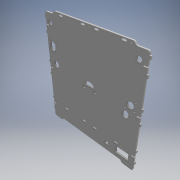
# Autodesk Inventor part: painel traseiro
Saved by Autodesk Inventor 2016 (Build 200138000, 138)
## iProperties
Created: 2016-08-08
Part Number: painel traseiro
Material: Generic
Document SubType Name: Modeling
Designer: Waldo
Density: 1 g/cm^3
Appearance: Default
Author: Waldo
Autodesk Inventor part; units mm, degrees
ref_plane "YZ Plane" through (0, 0, 0) normal (1, 0, 0) x (0, 1, 0)
ref_plane "XZ Plane" through (0, 0, 0) normal (0, 1, 0) x (-1, 0, 0)
ref_plane "XY Plane" through (0, 0, 0) normal (0, 0, 1) x (1, 0, 0)
sketch "Sketch1" plane through (0, 0, 0) normal (0, 1, 0) x (-1, 0, 0)
  line L0 (85.8953, -106.3896) -> (75.8953, -106.3896)
  line L1 (75.8953, -112.5896) -> (85.8953, -112.5896)
  line L2 (-145.1047, -106.3896) -> (-155.1047, -106.3896)
  line L3 (-155.1047, -112.5896) -> (-145.1047, -112.5896)
  line L4 (-54.6047, -106.3896) -> (-64.6047, -106.3896)
  line L5 (-64.6047, -112.5896) -> (-54.6047, -112.5896)
  line L6 (-4.6047, -106.3896) -> (-14.6047, -106.3896)
  line L7 (-14.6047, -112.5896) -> (-4.6047, -112.5896)
  line L8 (85.8953, 235.6104) -> (75.8953, 235.6104)
  line L9 (75.8953, 229.4104) -> (85.8953, 229.4104)
  line L10 (-145.1047, 235.6104) -> (-155.1047, 235.6104)
  line L11 (-155.1047, 229.4104) -> (-145.1047, 229.4104)
  line L12 (-54.6047, 235.6104) -> (-64.6047, 235.6104)
  line L13 (-64.6047, 229.4104) -> (-54.6047, 229.4104)
  line L14 (-4.6047, 235.6104) -> (-14.6047, 235.6104)
  line L15 (-14.6047, 229.4104) -> (-4.6047, 229.4104)
  line L16 (153.7371, 188.86) -> (147.2451, 188.86)
  line L17 (153.7371, 205.76) -> (153.7371, 188.86)
  line L18 (157.8955, 207.3098) -> (155.2869, 207.3098)
  line L19 (157.8955, 217.3104) -> (157.8955, 207.3098)
  line L20 (155.2869, 217.3104) -> (157.8955, 217.3104)
  line L21 (153.7371, 223.1102) -> (153.7371, 218.8602)
  line L22 (121.7453, 229.1102) -> (147.7371, 229.1102)
  line L23 (112.0224, 235.9739) -> (115.234, 232.1465)
  line L24 (105.511, 239.0102) -> (-174.7203, 239.0102)
  line L25 (-181.2317, 235.9739) -> (-184.4433, 232.1465)
  line L26 (-190.9547, 229.1102) -> (-216.9547, 229.1102)
  line L27 (-222.9547, 223.1102) -> (-222.9547, 218.8602)
  line L28 (-224.5045, 217.3104) -> (-227.1045, 217.3104)
  line L29 (-227.1045, 217.3104) -> (-227.1045, 207.3098)
  line L30 (-227.1045, 207.3098) -> (-224.5045, 207.3098)
  line L31 (-222.9547, 205.76) -> (-222.9547, 188.86)
  line L32 (-216.4542, 188.86) -> (-222.9547, 188.86)
  line L33 (-213.3942, 190.0596) -> (-214.9445, 190.0596)
  line L34 (-211.8813, 188.6771) -> (-211.8813, 188.8463)
  line L35 (-211.8813, 185.7741) -> (-211.8813, 185.9434)
  line L36 (-214.9445, 184.5607) -> (-213.3942, 184.5607)
  line L37 (-222.9547, 185.7604) -> (-216.4542, 185.7604)
  line L38 (-222.9547, 185.7604) -> (-222.9547, 168.8609)
  line L39 (-227.1127, 167.3111) -> (-224.5045, 167.3111)
  line L40 (-227.1127, 157.3107) -> (-227.1127, 167.3111)
  line L41 (-224.5045, 157.3107) -> (-227.1127, 157.3107)
  line L42 (-222.9547, 155.7609) -> (-222.9547, 65.5609)
  line L43 (-224.5045, 64.0111) -> (-227.1045, 64.0111)
  line L44 (-227.1045, 64.0111) -> (-227.1045, 54.0107)
  line L45 (-227.1045, 54.0107) -> (-224.5045, 54.0107)
  line L46 (-222.9547, 35.5607) -> (-222.9547, 52.4609)
  line L47 (-216.4542, 35.5607) -> (-222.9547, 35.5607)
  line L48 (-213.3942, 36.7603) -> (-214.9445, 36.7603)
  line L49 (-211.8813, 35.3778) -> (-211.8813, 35.547)
  line L50 (-211.8813, 32.4748) -> (-211.8813, 32.6441)
  line L51 (-214.9445, 31.2614) -> (-213.3942, 31.2614)
  line L52 (-222.9547, 32.4611) -> (-216.4542, 32.4611)
  line L53 (-222.9547, 15.5609) -> (-222.9547, 32.4611)
  line L54 (-227.1045, 14.0111) -> (-224.5045, 14.0111)
  line L55 (-227.1045, 4.0107) -> (-227.1045, 14.0111)
  line L56 (-224.5045, 4.0107) -> (-227.1045, 4.0107)
  line L57 (-222.9547, 2.4609) -> (-222.9547, -87.7398)
  line L58 (-224.5045, -89.2896) -> (-227.1045, -89.2896)
  line L59 (-227.1045, -89.2896) -> (-227.1045, -99.29)
  line L60 (-227.1045, -99.29) -> (-224.5045, -99.29)
  line L61 (-222.9547, -117.74) -> (-222.9547, -100.8398)
  line L62 (-216.4542, -117.74) -> (-222.9547, -117.74)
  line L63 (-213.3942, -116.5404) -> (-214.9445, -116.5404)
  line L64 (-211.8813, -117.9229) -> (-211.8813, -117.7537)
  line L65 (-211.8813, -120.8259) -> (-211.8813, -120.6566)
  line L66 (-214.9445, -122.0393) -> (-213.3942, -122.0393)
  line L67 (-222.9547, -120.8396) -> (-216.4542, -120.8396)
  line L68 (-222.9547, -137.7398) -> (-222.9547, -120.8396)
  line L69 (-227.1045, -139.2896) -> (-224.5045, -139.2896)
  line L70 (-227.1045, -149.29) -> (-227.1045, -139.2896)
  line L71 (-224.5045, -149.29) -> (-227.1045, -149.29)
  line L72 (-222.9547, -150.8398) -> (-222.9547, -174.9898)
  line L73 (-216.9547, -180.9898) -> (-184.9547, -180.9898)
  line L74 (-178.4433, -177.9535) -> (-174.2511, -172.9575)
  line L75 (100.8221, -170.9898) -> (-170.0314, -170.9898)
  line L76 (109.234, -177.9535) -> (105.0418, -172.9575)
  line L77 (147.7371, -180.9898) -> (115.7453, -180.9898)
  line L78 (153.7371, -150.8398) -> (153.7371, -174.9898)
  line L79 (155.2869, -149.29) -> (157.8955, -149.29)
  line L80 (157.8955, -149.29) -> (157.8955, -139.2896)
  line L81 (157.8955, -139.2896) -> (155.2869, -139.2896)
  line L82 (153.7371, -137.7398) -> (153.7371, -120.8396)
  line L83 (147.2451, -120.8396) -> (153.7371, -120.8396)
  line L84 (144.1849, -122.0393) -> (145.7353, -122.0393)
  line L85 (142.672, -120.6566) -> (142.672, -120.8259)
  line L86 (142.672, -117.7537) -> (142.672, -117.9229)
  line L87 (145.7354, -116.5404) -> (144.1849, -116.5404)
  line L88 (153.7371, -117.74) -> (147.2451, -117.74)
  line L89 (153.7371, -117.74) -> (153.7371, -100.8398)
  line L90 (157.8955, -99.29) -> (155.2869, -99.29)
  line L91 (157.8955, -89.2896) -> (157.8955, -99.29)
  line L92 (155.2869, -89.2896) -> (157.8955, -89.2896)
  line L93 (153.7371, 2.4609) -> (153.7371, -87.7398)
  line L94 (155.2869, 4.0107) -> (157.8955, 4.0107)
  line L95 (157.8955, 4.0107) -> (157.8955, 14.0111)
  line L96 (157.8955, 14.0111) -> (155.2869, 14.0111)
  line L97 (153.7371, 15.5609) -> (153.7371, 32.4611)
  line L98 (147.2451, 32.4611) -> (153.7371, 32.4611)
  line L99 (144.1849, 31.2614) -> (145.7353, 31.2614)
  line L100 (142.672, 32.6441) -> (142.672, 32.4748)
  line L101 (142.672, 35.547) -> (142.672, 35.3778)
  line L102 (145.7354, 36.7603) -> (144.1849, 36.7603)
  line L103 (153.7371, 35.5607) -> (147.2451, 35.5607)
  line L104 (153.7371, 35.5607) -> (153.7371, 52.4609)
  line L105 (157.8873, 54.0107) -> (155.2869, 54.0107)
  line L106 (157.8873, 64.0111) -> (157.8873, 54.0107)
  line L107 (155.2869, 64.0111) -> (157.8873, 64.0111)
  line L108 (153.7371, 155.7609) -> (153.7371, 65.5609)
  line L109 (155.2869, 157.3107) -> (157.8873, 157.3107)
  line L110 (157.8873, 157.3107) -> (157.8873, 167.3111)
  line L111 (157.8873, 167.3111) -> (155.2869, 167.3111)
  line L112 (153.7371, 185.7604) -> (153.7371, 168.8609)
  line L113 (147.2451, 185.7604) -> (153.7371, 185.7604)
  line L114 (144.1849, 184.5607) -> (145.7353, 184.5607)
  line L115 (142.672, 185.9434) -> (142.672, 185.7741)
  line L116 (142.672, 188.8463) -> (142.672, 188.6771)
  line L117 (145.7354, 190.0596) -> (144.1849, 190.0596)
  line L118 (142.672, 116.1611) -> (142.672, 124.6104)
  line L119 (118.1195, 124.4678) -> (118.2177, 116.019)
  line L120 (144.2572, 100.6103) -> (144.2572, 109.1103)
  line L121 (147.564, 109.1103) -> (147.564, 100.6103)
  line L122 (113.2572, 100.6103) -> (113.2572, 109.1103)
  line L123 (116.564, 109.1103) -> (116.564, 100.6103)
  line L124 (144.2593, 131.6103) -> (144.2593, 140.1103)
  line L125 (147.5662, 140.1103) -> (147.5662, 131.6103)
  line L126 (113.2593, 131.6103) -> (113.2593, 140.1103)
  line L127 (116.5662, 140.1103) -> (116.5662, 131.6103)
  line L128 (-58.5298, 26.7768) -> (-55.3303, 26.7768)
  line L129 (-55.6942, 39.6934) -> (-58.8457, 39.6934)
  line L130 (-13.5157, 39.6934) -> (-10.3641, 39.6934)
  line L131 (-10.68, 26.7768) -> (-13.8795, 26.7768)
  line L132 (-118.9547, -132.8214) -> (-106.9547, -132.8214)
  line L133 (-106.9547, -132.8214) -> (-106.9547, -144.8214)
  line L134 (-118.9547, -144.8214) -> (-106.9547, -144.8214)
  line L135 (-118.9547, -132.8214) -> (-118.9547, -144.8214)
  line L136 (-200.9547, -123.9896) -> (-152.9547, -123.9896)
  line L137 (-152.9547, -123.9896) -> (-152.9547, -151.9896)
  line L138 (-200.9547, -151.9896) -> (-152.9547, -151.9896)
  line L139 (-200.9547, -123.9896) -> (-200.9547, -151.9896)
  line L140 (-16.8277, 45.3022) -> (-17.455, 52.4764)
  line L141 (-50.8386, 43.6174) -> (-18.3716, 43.6174)
  line L142 (-51.7548, 52.4764) -> (-52.3825, 45.3023)
  line L143 (-185.1047, 15.6104) -> (-185.1047, 21.6104)
  line L144 (-165.1047, 21.6104) -> (-165.1047, 15.6104)
  circle A0 centre (-15.4247, 147.2638) radius 1.5
  circle A1 centre (-53.7847, 147.2638) radius 1.5
  circle A2 centre (131.8953, 198.6104) radius 8
  circle A3 centre (-197.9547, 198.6104) radius 8
  arc A4 (75.8953, -106.3896) -> (75.8953, -112.5896) centre (75.8953, -109.4896) ccw
  arc A5 (85.8953, -112.5896) -> (85.8953, -106.3896) centre (85.8953, -109.4896) ccw
  arc A6 (-155.1047, -106.3896) -> (-155.1047, -112.5896) centre (-155.1047, -109.4896) ccw
  arc A7 (-145.1047, -112.5896) -> (-145.1047, -106.3896) centre (-145.1047, -109.4896) ccw
  arc A8 (-64.6047, -106.3896) -> (-64.6047, -112.5896) centre (-64.6047, -109.4896) ccw
  arc A9 (-54.6047, -112.5896) -> (-54.6047, -106.3896) centre (-54.6047, -109.4896) ccw
  arc A10 (-14.6047, -106.3896) -> (-14.6047, -112.5896) centre (-14.6047, -109.4896) ccw
  arc A11 (-4.6047, -112.5896) -> (-4.6047, -106.3896) centre (-4.6047, -109.4896) ccw
  arc A12 (75.8953, 235.6104) -> (75.8953, 229.4104) centre (75.8953, 232.5104) ccw
  arc A13 (85.8953, 229.4104) -> (85.8953, 235.6104) centre (85.8953, 232.5104) ccw
  arc A14 (-155.1047, 235.6104) -> (-155.1047, 229.4104) centre (-155.1047, 232.5104) ccw
  arc A15 (-145.1047, 229.4104) -> (-145.1047, 235.6104) centre (-145.1047, 232.5104) ccw
  arc A16 (-64.6047, 235.6104) -> (-64.6047, 229.4104) centre (-64.6047, 232.5104) ccw
  arc A17 (-54.6047, 229.4104) -> (-54.6047, 235.6104) centre (-54.6047, 232.5104) ccw
  arc A18 (-14.6047, 235.6104) -> (-14.6047, 229.4104) centre (-14.6047, 232.5104) ccw
  arc A19 (-4.6047, 229.4104) -> (-4.6047, 235.6104) centre (-4.6047, 232.5104) ccw
  arc A20 (155.2869, 207.3098) -> (153.7371, 205.76) centre (155.2869, 205.76) ccw
  arc A21 (153.7371, 218.8602) -> (155.2869, 217.3104) centre (155.2869, 218.8602) ccw
  arc A22 (153.7371, 223.1102) -> (147.7371, 229.1102) centre (147.7371, 223.1102) ccw
  arc A23 (115.234, 232.1465) -> (121.7453, 229.1102) centre (121.7453, 237.6102) ccw
  arc A24 (112.0224, 235.9739) -> (105.511, 239.0102) centre (105.511, 230.5102) ccw
  arc A25 (-174.7203, 239.0102) -> (-181.2317, 235.9739) centre (-174.7203, 230.5102) ccw
  arc A26 (-190.9547, 229.1102) -> (-184.4433, 232.1465) centre (-190.9547, 237.6102) ccw
  arc A27 (-216.9547, 229.1102) -> (-222.9547, 223.1102) centre (-216.9547, 223.1102) ccw
  arc A28 (-224.5045, 217.3104) -> (-222.9547, 218.8602) centre (-224.5045, 218.8602) ccw
  arc A29 (-222.9547, 205.76) -> (-224.5045, 207.3098) centre (-224.5045, 205.76) ccw
  arc A30 (-214.9445, 190.0596) -> (-216.4542, 188.86) centre (-214.9445, 188.5098) ccw
  arc A31 (-211.8813, 188.8463) -> (-213.3942, 190.0596) centre (-213.3942, 188.5098) ccw
  arc A32 (-211.8813, 185.9434) -> (-211.8813, 188.6771) centre (-212.6118, 187.3102) ccw
  arc A33 (-213.3942, 184.5607) -> (-211.8813, 185.7741) centre (-213.3942, 186.1105) ccw
  arc A34 (-216.4542, 185.7604) -> (-214.9445, 184.5607) centre (-214.9445, 186.1105) ccw
  arc A35 (-224.5045, 167.3111) -> (-222.9547, 168.8609) centre (-224.5045, 168.8609) ccw
  arc A36 (-222.9547, 155.7609) -> (-224.5045, 157.3107) centre (-224.5045, 155.7609) ccw
  arc A37 (-224.5045, 64.0111) -> (-222.9547, 65.5609) centre (-224.5045, 65.5609) ccw
  arc A38 (-222.9547, 52.4609) -> (-224.5045, 54.0107) centre (-224.5045, 52.4609) ccw
  arc A39 (-214.9445, 36.7603) -> (-216.4542, 35.5607) centre (-214.9445, 35.2105) ccw
  arc A40 (-211.8813, 35.547) -> (-213.3942, 36.7603) centre (-213.3942, 35.2105) ccw
  arc A41 (-211.8813, 32.6441) -> (-211.8813, 35.3778) centre (-212.6118, 34.0109) ccw
  arc A42 (-213.3942, 31.2614) -> (-211.8813, 32.4748) centre (-213.3942, 32.8112) ccw
  arc A43 (-216.4542, 32.4611) -> (-214.9445, 31.2614) centre (-214.9445, 32.8112) ccw
  arc A44 (-224.5045, 14.0111) -> (-222.9547, 15.5609) centre (-224.5045, 15.5609) ccw
  arc A45 (-222.9547, 2.4609) -> (-224.5045, 4.0107) centre (-224.5045, 2.4609) ccw
  arc A46 (-224.5045, -89.2896) -> (-222.9547, -87.7398) centre (-224.5045, -87.7398) ccw
  arc A47 (-222.9547, -100.8398) -> (-224.5045, -99.29) centre (-224.5045, -100.8398) ccw
  arc A48 (-214.9445, -116.5404) -> (-216.4542, -117.74) centre (-214.9445, -118.0902) ccw
  arc A49 (-211.8813, -117.7537) -> (-213.3942, -116.5404) centre (-213.3942, -118.0902) ccw
  arc A50 (-211.8813, -120.6566) -> (-211.8813, -117.9229) centre (-212.6118, -119.2898) ccw
  arc A51 (-213.3942, -122.0393) -> (-211.8813, -120.8259) centre (-213.3942, -120.4895) ccw
  arc A52 (-216.4542, -120.8396) -> (-214.9445, -122.0393) centre (-214.9445, -120.4895) ccw
  arc A53 (-224.5045, -139.2896) -> (-222.9547, -137.7398) centre (-224.5045, -137.7398) ccw
  arc A54 (-222.9547, -150.8398) -> (-224.5045, -149.29) centre (-224.5045, -150.8398) ccw
  arc A55 (-222.9547, -174.9898) -> (-216.9547, -180.9898) centre (-216.9547, -174.9898) ccw
  arc A56 (-184.9547, -180.9898) -> (-178.4433, -177.9535) centre (-184.9547, -172.4898) ccw
  arc A57 (-170.0314, -170.9898) -> (-174.2511, -172.9575) centre (-170.0314, -176.4982) ccw
  arc A58 (105.0418, -172.9575) -> (100.8221, -170.9898) centre (100.8221, -176.4982) ccw
  arc A59 (109.234, -177.9535) -> (115.7453, -180.9898) centre (115.7453, -172.4898) ccw
  arc A60 (147.7371, -180.9898) -> (153.7371, -174.9898) centre (147.7371, -174.9898) ccw
  arc A61 (155.2869, -149.29) -> (153.7371, -150.8398) centre (155.2869, -150.8398) ccw
  arc A62 (153.7371, -137.7398) -> (155.2869, -139.2896) centre (155.2869, -137.7398) ccw
  arc A63 (145.7353, -122.0393) -> (147.2451, -120.8396) centre (145.7353, -120.4895) ccw
  arc A64 (142.672, -120.8259) -> (144.1849, -122.0393) centre (144.1849, -120.4895) ccw
  arc A65 (142.672, -117.9229) -> (142.672, -120.6566) centre (143.4025, -119.2898) ccw
  arc A66 (144.1849, -116.5404) -> (142.672, -117.7537) centre (144.1849, -118.0902) ccw
  arc A67 (147.2451, -117.74) -> (145.7354, -116.5404) centre (145.7354, -118.0902) ccw
  arc A68 (155.2869, -99.29) -> (153.7371, -100.8398) centre (155.2869, -100.8398) ccw
  arc A69 (153.7371, -87.7398) -> (155.2869, -89.2896) centre (155.2869, -87.7398) ccw
  arc A70 (155.2869, 4.0107) -> (153.7371, 2.4609) centre (155.2869, 2.4609) ccw
  arc A71 (153.7371, 15.5609) -> (155.2869, 14.0111) centre (155.2869, 15.5609) ccw
  arc A72 (145.7353, 31.2614) -> (147.2451, 32.4611) centre (145.7353, 32.8112) ccw
  arc A73 (142.672, 32.4748) -> (144.1849, 31.2614) centre (144.1849, 32.8112) ccw
  arc A74 (142.672, 35.3778) -> (142.672, 32.6441) centre (143.4025, 34.0109) ccw
  arc A75 (144.1849, 36.7603) -> (142.672, 35.547) centre (144.1849, 35.2105) ccw
  arc A76 (147.2451, 35.5607) -> (145.7354, 36.7603) centre (145.7354, 35.2105) ccw
  arc A77 (155.2869, 54.0107) -> (153.7371, 52.4609) centre (155.2869, 52.4609) ccw
  arc A78 (153.7371, 65.5609) -> (155.2869, 64.0111) centre (155.2869, 65.5609) ccw
  arc A79 (155.2869, 157.3107) -> (153.7371, 155.7609) centre (155.2869, 155.7609) ccw
  arc A80 (153.7371, 168.8609) -> (155.2869, 167.3111) centre (155.2869, 168.8609) ccw
  arc A81 (145.7353, 184.5607) -> (147.2451, 185.7604) centre (145.7353, 186.1105) ccw
  arc A82 (142.672, 185.7741) -> (144.1849, 184.5607) centre (144.1849, 186.1105) ccw
  arc A83 (142.672, 188.6771) -> (142.672, 185.9434) centre (143.4025, 187.3102) ccw
  arc A84 (144.1849, 190.0596) -> (142.672, 188.8463) centre (144.1849, 188.5098) ccw
  arc A85 (147.2451, 188.86) -> (145.7354, 190.0596) centre (145.7354, 188.5098) ccw
  arc A86 (142.672, 124.6104) -> (118.1195, 124.4678) centre (130.3953, 124.6104) ccw
  arc A87 (118.2177, 116.019) -> (142.672, 116.1611) centre (130.4444, 116.1611) ccw
  circle A88 centre (-170.9547, -110.9896) radius 1.6
  circle A89 centre (134.8196, 73.6104) radius 1.6
  arc A90 (144.2572, 100.6103) -> (147.564, 100.6103) centre (145.9106, 100.6103) ccw
  arc A91 (147.564, 109.1103) -> (144.2572, 109.1103) centre (145.9106, 109.1103) ccw
  arc A92 (113.2572, 100.6103) -> (116.564, 100.6103) centre (114.9106, 100.6103) ccw
  arc A93 (116.564, 109.1103) -> (113.2572, 109.1103) centre (114.9106, 109.1103) ccw
  arc A94 (144.2593, 131.6103) -> (147.5662, 131.6103) centre (145.9128, 131.6103) ccw
  arc A95 (147.5662, 140.1103) -> (144.2593, 140.1103) centre (145.9128, 140.1103) ccw
  arc A96 (113.2593, 131.6103) -> (116.5662, 131.6103) centre (114.9128, 131.6103) ccw
  arc A97 (116.5662, 140.1103) -> (113.2593, 140.1103) centre (114.9128, 140.1103) ccw
  circle A98 centre (134.8196, 42.6104) radius 1.6
  circle A99 centre (101.7453, -110.9896) radius 1.6
  circle A100 centre (-34.6047, 231.0104) radius 1.6
  arc A101 (-54.1733, 37.8455) -> (-55.6942, 39.6934) centre (-55.6942, 38.1436) ccw
  arc A102 (-54.1733, 37.8455) -> (-53.8357, 28.7365) centre (-34.6049, 34.0101) ccw
  arc A103 (-55.3303, 26.7768) -> (-53.8357, 28.7365) centre (-55.3303, 28.3266) ccw
  arc A104 (-60.0377, 27.9684) -> (-58.5298, 26.7768) centre (-58.5298, 28.3266) ccw
  arc A105 (-60.3735, 38.4041) -> (-60.0377, 27.9684) centre (-34.6049, 34.0101) ccw
  arc A106 (-58.8457, 39.6934) -> (-60.3735, 38.4041) centre (-58.8457, 38.1436) ccw
  arc A107 (-8.8364, 38.4041) -> (-10.3641, 39.6934) centre (-10.3641, 38.1436) ccw
  arc A108 (-9.1722, 27.9684) -> (-8.8364, 38.4041) centre (-34.6049, 34.0101) ccw
  arc A109 (-10.68, 26.7768) -> (-9.1722, 27.9684) centre (-10.68, 28.3266) ccw
  arc A110 (-15.3742, 28.7365) -> (-13.8795, 26.7768) centre (-13.8795, 28.3266) ccw
  arc A111 (-15.3742, 28.7365) -> (-15.0365, 37.8455) centre (-34.6049, 34.0101) ccw
  arc A112 (-13.5157, 39.6934) -> (-15.0365, 37.8455) centre (-13.5157, 38.1436) ccw
  arc A113 (-17.455, 52.4764) -> (-17.9943, 53.5214) centre (-18.9989, 52.3414) ccw
  arc A114 (-18.3716, 43.6174) -> (-16.8277, 45.3022) centre (-18.3716, 45.1672) ccw
  arc A115 (-52.3825, 45.3023) -> (-50.8386, 43.6174) centre (-50.8386, 45.1672) ccw
  arc A116 (-51.2156, 53.5214) -> (-51.7548, 52.4764) centre (-50.2109, 52.3414) ccw
  arc A117 (-17.9943, 53.5214) -> (-51.2156, 53.5214) centre (-34.6049, 34.0101) ccw
  circle A118 centre (101.7453, 231.0104) radius 1.6
  circle A119 centre (-177.5547, -117.9896) radius 1.5
  circle A120 centre (-176.3547, -157.9896) radius 1.5
  circle A121 centre (-188.1047, 57.6104) radius 11.5
  circle A122 centre (-204.0289, 73.6104) radius 1.6
  circle A123 centre (-173.0289, 73.6104) radius 1.6
  circle A124 centre (-204.0289, 42.6104) radius 1.6
  circle A125 centre (-173.0289, 42.6104) radius 1.6
  arc A126 (-185.1047, 15.6104) -> (-165.1047, 15.6104) centre (-175.1047, 15.6104) ccw
  arc A127 (-165.1047, 21.6104) -> (-185.1047, 21.6104) centre (-175.1047, 21.6104) ccw
  circle A128 centre (-127.9547, -137.9896) radius 1.5
  circle A129 centre (-170.9547, 231.0104) radius 1.6
  circle A130 centre (-97.9547, -137.9896) radius 1.5
  circle A131 centre (103.8196, 42.6104) radius 1.6
  circle A132 centre (103.8196, 73.6104) radius 1.6
  circle A133 centre (118.8953, 57.6104) radius 11.5
  circle A134 centre (-197.9547, 198.6104) radius 4
  circle A135 centre (131.8953, 198.6104) radius 4
  point P0 (0, 0)
  constraints: 310 tangent, 290 end point, 222 point on circle, 136 centre point, 95 equal radius, 67 parallel, 20 perpendicular, 1 collinear
extrude "Extrusion1" add sketch "Sketch1" along normal blind 6 contours L16 A85 L117 A84 L116 A83 L115 A82 L114 A81 L113 L112 A80 L111 L110 L109 A79 L108 A78 L107 L106 L105 A77 L104 L103 A76 L102 A75 L101 A74 L100 A73 L99 A72 L98 L97 A71 L96 L95 L94 A70 L93 A69 L92 L91 L90 A68 L89 L88 A67 L87 A66 L86 A65 L85 A64 L84 A63 L83 L82 A62 L81 L80 L79 A61 L78 A60 L77 A59 L76 A58 L75 A57 L74 A56 L73 A55 L72 A54 L71 L70 L69 A53 L68 L67 A52 L66 A51 L65 A50 L64 A49 L63 A48 L62 L61 A47 L60 L59 L58 A46 L57 A45 L56 L55 L54 A44 L53 L52 A43 L51 A42 L50 A41 L49 A40 L48 A39 L47 L46 A38 L45 L44 L43 A37 L42 A36 L41 L40 L39 A35 L38 L37 A34 L36 A33 L35 A32 L34 A31 L33 A30 L32 L31 A29 L30 L29 L28 A28 L27 A27 L26 A26 L25 A25 L24 A24 L23 A23 L22 A22 L21 A21 L20 L19 L18 A20 L17
body "Solid1"
